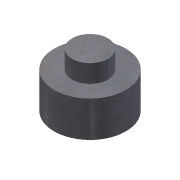
# Autodesk Inventor part: roll2
Saved by Autodesk Inventor 2022 (Build 260148000, 148)
## iProperties
Shininess: 64.0
Length Units: 11269
Angle Units: 11279
Time Units: 11290
Mass Units: 11283
Length Display Precision: 3
Angle Display Precision: 2
Created: 2001-12-31
Part Number: roll2
Document SubType Name: Modeling
Designer: Administrator
Density: 1 g/cm^3
Material: Generic
Appearance: Oxidized
Density: 0.0
Volumn: 0.0
Area: 0.0
PropertySet Name: Model Information
Control State: 0
Master: False
Checked Out: False
Author: Administrator
Autodesk Inventor part; units mm, degrees
ref_plane "YZ Plane" through (0, 0, 0) normal (1, 0, 0) x (0, 1, 0)
ref_plane "XZ Plane" through (0, 0, 0) normal (0, 1, 0) x (-1, 0, 0)
ref_plane "XY Plane" through (0, 0, 0) normal (0, 0, 1) x (1, 0, 0)
sketch "Sketch1" plane through (0, 0, 0) normal (0, 0, 1) x (1, 0, 0)
  line L0 (-8.1504, 12.0476) -> (-8.1504, 5.6976)
  line L1 (-8.1504, 5.6976) -> (-14.5004, 5.6976)
  line L2 (-14.5004, 5.6976) -> (-14.5004, -7.0024)
  line L3 (-14.5004, -7.0024) -> (-3.0704, -7.0024)
  line L4 (-3.0704, -7.0024) -> (-3.0704, -13.3524)
  line L5 (-3.0704, -13.3524) -> (-1.8004, -13.3524)
  line L6 (-1.8004, 12.0476) -> (-8.1504, 12.0476)
  line L7 (-1.8004, 12.0476) -> (-1.8004, -13.3524)
  dimension "d0" = 12.7
  dimension "d1" = 6.35
  dimension "d3" = 1.27
  dimension "d8" = 12.7
  dimension "d9" = 6.35
  constraints: 16 end point, 5 parallel, 2 vertical, 1 perpendicular
  measures "d0" distance of L1.end L2.end
  measures "d1" distance of L0.start L0.end
  measures "d3" distance of L4.end L5.end
  measures "d8" horizontal distance of L2.end L5.end
  measures "d9" distance of L6.start L0.start
revolve "Revolution1" add sketch "Sketch1" angle 360 about axis through (-1.8004, 12.0476, 0) along (0, -1, 0)
body "Solid1"
